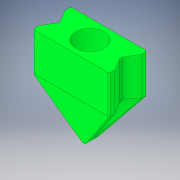
# Autodesk Inventor part: Selector
Saved by Autodesk Inventor 2018.1 (Build 221171000, 171)
## iProperties
Created: 2017-12-03
Part Number: Selector
Material: Generic
Document SubType Name: Modeling
Designer: xdlea
Density: 1 g/cm^3
Appearance: Default(1)
Author: xdlea
Autodesk Inventor part; units mm, degrees
ref_plane "YZ Plane" through (0, 0, 0) normal (1, 0, 0) x (0, 1, 0)
ref_plane "XZ Plane" through (0, 0, 0) normal (0, 1, 0) x (-1, 0, 0)
sketch "Sketch1" plane through (0, 0, 0) normal (0, 0, 1) x (1, 0, 0)
  line L0 (-6.35, -3.175) -> (6.35, -3.175) construction
  line L1 (6.35, -3.175) -> (6.35, 3.175)
  line L2 (6.35, 3.175) -> (-6.35, 3.175)
  line L3 (-6.35, 3.175) -> (-6.35, -3.175)
  line L4 (-6.35, -3.175) -> (6.35, 3.175) construction
  line L5 (6.35, -3.175) -> (-6.35, 3.175) construction
  line L6 (0, 6.0606) -> (0, -14.1385) construction
  line L7 (-6.35, -3.175) -> (-0.3234, -11.0927)
  line L8 (6.35, -3.175) -> (0.3234, -11.0927)
  arc A0 (-0.3234, -11.0927) -> (0.3234, -11.0927) centre (0, -10.8466) ccw
  point P0 (0, 0)
  dimension "d0" = 12.7
  dimension "d1" = 6.35
  dimension "d3" = 0.4064
  constraints: 16 end point, 2 midpoint, 2 parallel, 2 point on circle, 2 tangent, 1 centre point, 1 horizontal, 1 perpendicular, 1 point on line
  measures "d0" distance of L1.end L2.end
  measures "d1" distance of L0.end L1.end
  measures "d3" radius of A0
extrude "Extrusion1" add sketch "Sketch1" along normal mid plane 6.35
sketch "Sketch2" plane through (0, 0, 0) normal (0, 0, 1) x (1, 0, 0)
  line L0 (6.35, -3.175) -> (6.35, 3.175) projected
  line L1 (-6.35, 3.175) -> (-6.35, -3.175) projected
  line L2 (-6.35, -3.175) -> (-0.3517, -13.5393)
  arc A0 (-0.3517, -13.5393) -> (0.3517, -13.5393) centre (0, -13.3358) ccw
  line L3 (6.35, -3.175) -> (0.3517, -13.5393)
  arc A1 (-0.3234, -11.0927) -> (0.3234, -11.0927) centre (0, -10.8466) ccw projected
  point P0 (0, 0)
  dimension "d9" = 0.4064
  dimension "d10" = 2.4892
  constraints: 4 end point, 2 point on circle, 2 tangent, 1 centre point, 1 vertical alignment
  measures "d9" radius of A0
  measures "d10" distance of A0.centre A1.centre
sketch "Sketch3" plane through (-6.35, 3.175, 3.175) normal (0, 1, 0) x (1, 0, 0)
  line L0 (12.7, 0.9525) -> (11.5177, 2.9571)
  line L1 (11.5177, 3.3929) -> (12.7, 5.3975)
  line L2 (12.7, 5.3975) -> (12.7, 0.9525)
  arc A0 (11.5177, 3.3929) -> (11.5177, 2.9571) centre (11.8872, 3.175) ccw
  line L3 (12.7, 3.175) -> (11.8872, 3.175) construction
  point P0 (6.35, 3.175)
  dimension "d7" = 0.429
  dimension "d13" = 4.445
  dimension "d14" = 0.8128
  constraints: 8 end point, 2 midpoint, 2 point on circle, 1 centre point, 1 horizontal alignment, 1 point on line, 1 tangent, 1 vertical, 1 other
  measures "d7" radius of A0
  measures "d13" distance of L1.end L0.start
  measures "d14" distance of L3.start L3.end
sweep "Sweep1" cut profiles "Sketch3" path "Sketch2" path curves L0 L3 A0 L2 L1
ref_plane "Work Plane2" through (6.35, -3.175, -3.175) normal (0, -0.2586, -0.966) x (-0.5924, -0.7783, 0.2083)
ref_plane "Work Plane1" through (3.1636, -7.3612, -1.1019) normal (0, -0.2586, -0.966) x (-0.5924, -0.7783, 0.2083)
sketch "Sketch4" plane through (6.35, -3.175, -3.175) normal (0, -0.2586, -0.966) x (-0.5924, -0.7783, 0.2083)
  line L0 (10.1736, 0) -> (0, 0) projected
  line L1 (0, 0) -> (7.5232, 10.2319) projected
  line L2 (7.5232, 10.2319) -> (10.5567, 0.5211) projected
  ellipse E0 centre (10.1599, 0.4115) end of major axis (9.8209, 0.6607) minor radius 0.4064 (10.1736, 0) -> (10.5567, 0.5211) ccw projected
  point P0 (1.9521, 6.4464)
  constraints: 1 other
extrude "Extrusion2" cut sketch "Sketch4" along normal up to next
mirror "Mirror1" about plane through (0, 0, 0) normal (0, 0, 1) of "Extrusion2"
chamfer "Chamfer1" distance 0.2032 angle 45 4 edges at (6.35, 0, -3.175) (6.35, 0, 3.175) (-6.35, 0, -3.175) (-6.35, 0, 3.175)
sketch "Sketch5" plane through (5.5372, 3.175, 0) normal (0, 1, 0) x (1, 0, 0)
  circle A0 centre (-5.5372, 0) radius 2.3813
  dimension "d20" = 4.7625
  constraints: 1 centre point, 1 coincident
  measures "d20" diameter of A0
extrude "Extrusion3" cut sketch "Sketch5" against normal blind 6.35
body "Solid1"
